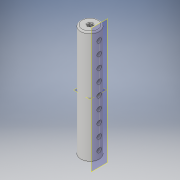
# Autodesk Inventor part: tube
Saved by Autodesk Inventor 2019 (Build 230136000, 136)
## iProperties
Created: 2018-09-29
Part Number: tube
Material: Generic
Document SubType Name: Modeling
Designer: mrhftc
Density: 1 g/cm^3
Appearance: Default
Author: mrhftc
Autodesk Inventor part; units mm, degrees
ref_plane "YZ Plane" through (0, 0, 0) normal (1, 0, 0) x (0, 1, 0)
ref_plane "XZ Plane" through (0, 0, 0) normal (0, 1, 0) x (-1, 0, 0)
ref_plane "XY Plane" through (0, 0, 0) normal (0, 0, 1) x (1, 0, 0)
sketch "Sketch3" plane through (0, 0, 0) normal (0, 1, 0) x (-1, 0, 0)
  circle A0 centre (0, 0) radius 12.5
  line L0 (0, 7.3639) -> (0, 0)
  line L1 (0, 0) -> (0, -8.8137)
  line L2 (6.485, 0) -> (0, 0)
  line L3 (-6.963, 0) -> (0, 0)
  line L4 (0, 3.0022) -> (2.6, 1.5011)
  line L5 (0, 3.0022) -> (3.0022, 3.0022) construction
  circle A1 centre (0, 0) radius 12.5
  line L6 (0, 3.0022) -> (-2.6, 1.5011)
  line L7 (0, -3.0022) -> (2.6, -1.5011)
  line L8 (0, -3.0022) -> (-2.6, -1.5011)
  line L9 (2.6, 1.5011) -> (2.6, -1.5011)
  line L10 (-2.6, 1.5011) -> (-2.6, -1.5011)
  dimension "d6" = 30
  dimension "d7" = 5.2
  dimension "d8" = 3.0022
  dimension "d9" = 3.0022
  dimension "d26" = 25
  constraints: 22 end point, 4 symmetric about line, 3 point on line, 2 centre point, 2 horizontal, 2 vertical, 1 coincident, 1 collinear, 1 equal length, 1 parallel, 1 other
  measures "d6" angle of L4 L5
  measures "d7" distance between parallel lines of L6 L7
  measures "d8" distance of L4.start L4.end
  measures "d9" distance of L4.end L7.end
  measures "d26" diameter of A0
extrude "Extrusion2" add sketch "Sketch3" along normal blind 152.4
fillet "Fillet3" radius 2 1 edges at (12.5, 0, 0)
fillet "Fillet4" radius 1 6 edges at (1.3, 0, -2.2517) (-1.3, 0, -2.2517) (-2.6, 0, 0) (-1.3, 0, 2.2517) (1.3, 0, 2.2517) (2.6, 0, 0)
ref_plane "Work Plane1" through (0, 76.2, 0) normal (0, -1, 0) x (1, 0, 0)
mirror "Mirror1" about plane through (0, 76.2, 0) normal (0, -1, 0) of "Fillet4", "Fillet3"
ref_plane "Work Plane2" through (12.5, 0, 0) normal (-1, 0, 0) x (0, -1, 0)
sketch "Sketch4" plane through (12.5, 0, 0) normal (-1, 0, 0) x (0, -1, 0)
  line L0 (-150.4, 12.5) -> (-150.4, -12.5) projected
  line L1 (-150.4, 0) -> (0, 0)
  line L2 (-1, 3.0022) -> (-151.4, 3.0022) projected
  circle A0 centre (-76.2, 0) radius 3
  circle A1 centre (-60.2, 0) radius 3
  circle A2 centre (-44.2, 0) radius 3
  circle A3 centre (-28.2, 0) radius 3
  circle A4 centre (-12.2, 0) radius 3
  circle A5 centre (-92.2, 0) radius 3
  circle A6 centre (-76.2, 0) radius 3
  circle A7 centre (-60.2, 0) radius 3
  circle A8 centre (-44.2, 0) radius 3
  circle A9 centre (-28.2, 0) radius 3
  circle A10 centre (-108.2, 0) radius 3
  circle A11 centre (-92.2, 0) radius 3
  circle A12 centre (-76.2, 0) radius 3
  circle A13 centre (-60.2, 0) radius 3
  circle A14 centre (-44.2, 0) radius 3
  circle A15 centre (-124.2, 0) radius 3
  circle A16 centre (-108.2, 0) radius 3
  circle A17 centre (-92.2, 0) radius 3
  circle A18 centre (-76.2, 0) radius 3
  circle A19 centre (-60.2, 0) radius 3
  circle A20 centre (-140.2, 0) radius 3
  circle A21 centre (-124.2, 0) radius 3
  circle A22 centre (-108.2, 0) radius 3
  circle A23 centre (-92.2, 0) radius 3
  circle A24 centre (-76.2, 0) radius 3
  dimension "d17" = 6
  dimension "d20" = 16
  dimension "d23" = 16
  constraints: 25 centre point, 2 end point, 2 horizontal, 1 midpoint, 1 parallel, 1 point on line, 48 other
  measures "d17" diameter of A0
  measures "d20" distance of A0.centre A1.centre
  measures "d23" distance of A0.centre A5.centre
extrude "Extrusion3" cut sketch "Sketch4" along normal blind 7
pattern_circular "Circular Pattern1" count 2 over 360 about axis through (0, 2, 0) along (0, -1, 0) of "Extrusion3"
equation "\"d8\" = d9"
body "Solid2"
